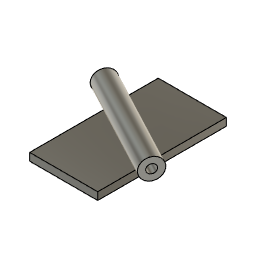
Pipe_Attached_to_a_Cuboid (Autodesk Fusion 360 design; units mm, degrees)
Autodesk Fusion 360 part; units mm, degrees
sketch "Rectangle" plane through (0, 0, 0) normal (0, 0, 1) x (1, 0, 0)
  line L0 (45, -85) -> (-45, -85)
  line L1 (-45, -85) -> (-45, 85)
  line L2 (-45, 85) -> (45, 85)
  line L3 (45, 85) -> (45, -85)
  line L4 (45, -85) -> (-45, 85) construction
  line L5 (-45, -85) -> (45, 85) construction
  constraint horizontal L0
  constraint perpendicular L0 L1
  constraint parallel L0 L2
  constraint parallel L1 L3
  constraint coincident L4 origin
  constraint coincident L5 origin
extrude "Extrude1" add sketch "Rectangle" along normal blind 10
sketch "Diagonals" plane through (0, 0, 10) normal (0, 0, 1) x (-1, 0, 0)
  line L0 (-45, -85) -> (45, -85)
  line L1 (45, -85) -> (45, 85)
  line L2 (45, 85) -> (-45, 85)
  line L3 (-45, 85) -> (-45, -85)
  line L4 (45, -85) -> (-45, 85) construction
  line L5 (-45, -85) -> (45, 85) construction
  line L6 (45, -23.8236) -> (-45, 23.8235)
  dimension "d3" = 90
  constraint coincident L0.end L1.start
  constraint coincident L2.end L3.start
  constraint coincident L0.start L3.end
  constraint coincident L1.end L2.start
  constraint coincident L1 L6.start
  constraint coincident L3 L6.end
  measures "d3" angle of L5 L6
ref_plane "WorkPlane1" through (0, 0, 10) normal (0.883788, -0.467888, 0) x (0.467888, 0.883788, 0)
sketch "Circles" plane through (0, 0, 10) normal (0.883788, -0.467888, 0) x (0.467888, 0.883788, 0)
  circle A0 centre (0, 12) radius 5.831
  circle A1 centre (0, 12) radius 13.9284
  constraint concentric A0 A1
extrude "Extrude2" add sketch "Circles" along normal mid plane 150
named bodies: "Pipe_Attached_to_a_Cuboid"
